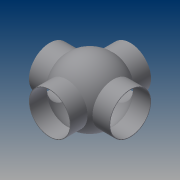
# Autodesk Inventor part: ISO_200_Cross_4way_Sphere
Saved by Autodesk Inventor 2015 SP1 (Build 190203100, 203)
## iProperties
Created: 2015-04-08
Part Number: ISO_200_Cross_4way_Sphere
Material: Generic
Document SubType Name: Modeling
Designer: nfitch
Density: 1 g/cm^3
Appearance: Default
Author: nfitch
Autodesk Inventor part; units mm, degrees
ref_plane "YZ Plane" through (0, 0, 0) normal (1, 0, 0) x (0, 1, 0)
ref_plane "XY Plane" through (0, 0, 0) normal (0, 0, 1) x (1, 0, 0)
sketch "Sketch1" plane through (0, 0, 0) normal (1, 0, 0) x (0, 1, 0)
  arc A0 (-152.4, 0) -> (152.4, 0) centre (0, 0) ccw
  arc A1 (-149.35, 0) -> (149.35, 0) centre (0, 0) ccw
  line L0 (152.4, 0) -> (149.35, 0)
  line L1 (-149.35, 0) -> (-152.4, 0)
  line L2 (-213.36, 0) -> (213.36, 0) projected
  dimension "d0" = 152.4
  dimension "d2" = 149.35
  constraints: 4 end point, 4 point on circle, 2 centre point, 1 coincident, 1 collinear, 1 horizontal
  measures "d0" radius of A0
  measures "d2" radius of A1
revolve "Revolution1" add sketch "Sketch1" angle 360 about axis through (0, -10, 0) along (0, 1, 0) contours L1 A1 L0 A0
sketch "Sketch2" plane through (0, 0, 0) normal (1, 0, 0) x (0, 1, 0)
  circle A0 centre (0, 0) radius 98.5
  dimension "d4" = 197
  constraints: 1 centre point, 1 coincident
  measures "d4" diameter of A0
extrude "Extrusion1" cut sketch "Sketch2" along normal through all both and the other way through all
sketch "Sketch3" plane through (0, 0, 0) normal (0, 1, 0) x (-1, 0, 0)
  circle A0 centre (0, 0) radius 98.5
  dimension "d7" = 197
  constraints: 1 centre point, 1 coincident
  measures "d7" diameter of A0
extrude "Extrusion2" cut sketch "Sketch3" along normal through all both and the other way through all
ref_plane "Work Plane1" through (0, 196.85, 0) normal (0, 1, 0) x (-1, 0, 0)
sketch "Sketch4" plane through (0, 196.85, 0) normal (0, 1, 0) x (-1, 0, 0)
  circle A0 centre (0, 0) radius 101.6
  circle A1 centre (0, 0) radius 98.5 projected
  circle A2 centre (0, 0) radius 98.5
  dimension "d11" = 203.2
  dimension "d12" = 197
  constraints: 2 centre point, 2 coincident
  measures "d11" diameter of A0
  measures "d12" diameter of A2
extrude "Extrusion3" add sketch "Sketch4" against normal up to next
pattern_circular "Circular Pattern1" count 4 over 360 about axis through (0, 0, -10) along (0, 0, 1) of "Extrusion3"
body "Solid1"
